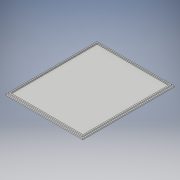
# Autodesk Inventor part: Lid
Saved by Autodesk Inventor 2019 (Build 230136000, 136)
## iProperties
Created: 2019-02-20
Part Number: Lid
Material: Generic
Document SubType Name: Modeling
Designer: Austin
Density: 1 g/cm^3
Appearance: Default
Author: Austin
Autodesk Inventor part; units mm, degrees
ref_plane "YZ Plane" through (0, 0, 0) normal (1, 0, 0) x (0, 1, 0)
ref_plane "XZ Plane" through (0, 0, 0) normal (0, 1, 0) x (-1, 0, 0)
ref_plane "XY Plane" through (0, 0, 0) normal (0, 0, 1) x (1, 0, 0)
sketch "Sketch1" plane through (0, 0, 0) normal (0, 1, 0) x (-1, 0, 0)
  line L0 (0, 0) -> (-171.45, 0)
  line L1 (-171.45, 0) -> (-171.45, -203.2)
  line L2 (-171.45, -203.2) -> (0, -203.2)
  line L3 (0, -203.2) -> (0, 0)
  dimension "d0" = 171.45
  dimension "d2" = 203.2
  constraints: 8 end point, 2 parallel, 1 horizontal, 1 perpendicular
  measures "d0" distance of L2.end L1.end
  measures "d2" distance of L1.end L0.end
extrude "Extrusion1" add sketch "Sketch1" against normal blind 2.54
sketch "Sketch4" plane through (0, -2.54, 0) normal (0, -1, 0) x (1, 0, 0)
  line L0 (168.91, -2.54) -> (2.54, -2.54)
  line L1 (2.54, -2.54) -> (2.54, -200.66)
  line L2 (2.54, -200.66) -> (168.91, -200.66)
  line L3 (168.91, -200.66) -> (168.91, -2.54)
  line L4 (171.45, 0) -> (171.45, -203.2) projected
  line L5 (171.45, -203.2) -> (0, -203.2) projected
  line L6 (0, 0) -> (171.45, 0) projected
  line L7 (0, -203.2) -> (0, 0) projected
  dimension "d20" = 2.54
  dimension "d21" = 2.54
  dimension "d22" = 2.54
  dimension "d23" = 2.54
  constraints: 8 end point, 2 parallel, 1 horizontal, 1 perpendicular
  measures "d20" distance between parallel lines of L3 L4
  measures "d21" distance between parallel lines of L2 L5
  measures "d22" distance between parallel lines of L6 L0
  measures "d23" distance between parallel lines of L7 L1
extrude "Extrusion3" add sketch "Sketch4" against normal blind 5.08 contours L3 L2 L1 L0
sketch "Sketch6" plane through (0, 2.54, 0) normal (0, 1, 0) x (1, 0, 0)
  line L0 (5.08, 5.08) -> (166.37, 5.08)
  line L1 (166.37, 5.08) -> (166.37, 198.12)
  line L2 (166.37, 198.12) -> (5.08, 198.12)
  line L3 (5.08, 198.12) -> (5.08, 5.08)
  line L4 (2.54, 200.66) -> (2.54, 2.54) projected
  line L5 (168.91, 200.66) -> (2.54, 200.66) projected
  line L6 (168.91, 2.54) -> (168.91, 200.66) projected
  line L7 (2.54, 2.54) -> (168.91, 2.54) projected
  point P0 (0, 0)
  dimension "d24" = 2.54
  dimension "d25" = 2.54
  dimension "d26" = 2.54
  dimension "d27" = 2.54
  constraints: 8 end point, 2 parallel, 1 horizontal, 1 perpendicular
  measures "d24" distance between parallel lines of L4 L3
  measures "d25" distance between parallel lines of L5 L2
  measures "d26" distance between parallel lines of L1 L6
  measures "d27" distance between parallel lines of L7 L0
extrude "Extrusion4" cut sketch "Sketch6" against normal blind 2.54 contours L3 L2 L1 L0
body "Solid1"
